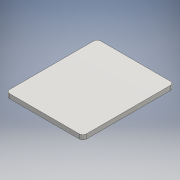
# Autodesk Inventor part: PerfBoard
Saved by Autodesk Inventor 2016 (Build 200138000, 138)
## iProperties
Created: 2016-05-01
Part Number: PerfBoard
Material: Generic
Document SubType Name: Modeling
Designer: Owner
Density: 1 g/cm^3
Appearance: White
Author: Owner
Autodesk Inventor part; units mm, degrees
ref_plane "YZ Plane" through (0, 0, 0) normal (1, 0, 0) x (0, 1, 0)
ref_plane "XZ Plane" through (0, 0, 0) normal (0, 1, 0) x (-1, 0, 0)
ref_plane "XY Plane" through (0, 0, 0) normal (0, 0, 1) x (1, 0, 0)
sketch "Sketch1" plane through (0, 0, 0) normal (0, 0, 1) x (1, 0, 0)
  line L0 (2, 0) -> (41, 0)
  line L1 (43, 2) -> (43, 49)
  line L2 (41, 51) -> (2, 51)
  line L3 (0, 49) -> (0, 2)
  arc A0 (2, 51) -> (0, 49) centre (2, 49) ccw
  arc A1 (0, 2) -> (2, 0) centre (2, 2) ccw
  arc A2 (41, 0) -> (43, 2) centre (41, 2) ccw
  arc A3 (43, 49) -> (41, 51) centre (41, 49) ccw
  point P0 (0, 0)
  point P1 (43, 51)
  point P2 (43, 0)
  dimension "d0" = 43
  dimension "d1" = 51
  dimension "d2" = 2
  dimension "d3" = 2
  constraints: 8 end point, 8 point on circle, 8 tangent, 6 point on line, 4 centre point, 2 equal radius, 2 parallel, 1 horizontal, 1 perpendicular
  measures "d0" distance of point (0, 0) point (43, 0)
  measures "d1" distance of point (43, 0) point (43, 51)
  measures "d2" radius of A0
  measures "d3" radius of A1
extrude "Extrusion1" add sketch "Sketch1" along normal blind 2.5
body "Solid1"
